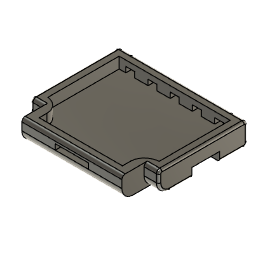
Carcasa Muñeca v1 (Autodesk Fusion 360 design; units mm, degrees)
Autodesk Fusion 360 part; units mm, degrees
sketch "Sketch10" plane through (0, 0, 0) normal (0, 0, 1) x (1, 0, 0)
  line L0 (0, -50) -> (0, 50) construction
  line L1 (0, 50) -> (-57, 50)
  line L2 (-57, 50) -> (-57, 0)
  line L3 (0, -50) -> (-45, -50)
  line L4 (-45, -50) -> (-45, -30)
  arc A0 (-57, 0) -> (-45, -30) centre (-7.0663, 2.5735) ccw
  line L5 (0, -50) -> (45, -50)
  line L6 (45, -50) -> (45, -30)
  arc A1 (45, -30) -> (57, 0) centre (7.0663, 2.5735) ccw
  line L7 (57, 50) -> (57, 0)
  line L8 (0, 50) -> (57, 50)
  dimension "d19" = 100
  dimension "d20" = 57
  dimension "d21" = 50
  dimension "d22" = 45
  dimension "d23" = 20
  dimension "d24" = 50
  dimension "d25" = 30
  constraint vertical L0
  constraint midpoint L0 origin
  constraint perpendicular L0 L1
  constraint perpendicular L1 L2
  constraint perpendicular L0 L3
  constraint perpendicular L3 L4
  constraint symmetric L3.start L0 L5.start
  constraint symmetric L1.start L0 L8.start
  constraint symmetric L0 L1.end L7.start
  constraint symmetric L0 L2.end A1.end
  constraint symmetric L0 L3.end L5.end
  constraint symmetric L0 L4.end L6.end
  constraint symmetric L0 A0 A1
  measures "d19" distance of L0.start L0.end
  measures "d20" distance of L0.end L1.end
  measures "d21" distance of L1.end L2.end
  measures "d22" distance of L0.start L3.end
  measures "d23" distance of L3.end L4.end
  measures "d24" radius of A0
  measures "d25" vertical distance of L2.end L4.end
sketch "Sketch12" plane through (0, 0, 0) normal (1, 0, 0) x (0, 1, 0)
  line L0 (0, 10) -> (0, -10) construction
  line L1 (0, 10) -> (47, 10)
  line L2 (50, 7) -> (50, -7)
  line L3 (47, -10) -> (0, -10)
  arc A0 (50, 7) -> (47, 10) centre (47, 7) ccw
  line L4 (0, 10) -> (-47, 10)
  line L5 (-50, 7) -> (-50, 0)
  line L6 (-40, -10) -> (0, -10)
  arc A1 (-47, 10) -> (-50, 7) centre (-47, 7) ccw
  arc A2 (-50, 0) -> (-40, -10) centre (-40, 0) ccw
  arc A3 (47, -10) -> (50, -7) centre (47, -7) ccw
  dimension "d30" = 3
  dimension "d31" = 47
  dimension "d34" = 3
  dimension "d35" = 10
  dimension "d36" = 7
  dimension "d37" = 40
  dimension "d38" = 3
  dimension "d39" = 47
  dimension "d40" = 14
  constraint vertical L0
  constraint midpoint L0 origin
  constraint perpendicular L0 L1
  constraint perpendicular L1 L2
  constraint tangent L1 A0
  constraint tangent L2 A0
  constraint perpendicular L0 L4
  constraint perpendicular L4 L5
  constraint tangent L5 A1
  constraint tangent L4 A1
  constraint tangent L6 A2
  constraint tangent L5 A2
  constraint tangent L3 A3
  constraint tangent L2 A3
  measures "d30" radius of A0
  measures "d31" distance of L0.start L1.end
  measures "d34" radius of A1
  measures "d35" radius of A2
  measures "d36" distance of L5.start L5.end
  measures "d37" distance of L0.end L6.start
  measures "d38" radius of A3
  measures "d39" distance of L0.end L3.start
  measures "d40" distance of L2.start L2.end
extrude "Extrude1" add sketch "Sketch12" along normal mid plane 90
ref_plane "WorkPlane5" through (-57, 0, 0) normal (-1, 0, 0) x (0, -1, 0)
sketch "Sketch14" plane through (-57, 0, 0) normal (-1, 0, 0) x (0, 1, 0)
ref_plane "WorkPlane6" through (-57, 25, 0) normal (-1, 0, 0) x (0, -1, 0)
sketch "Sketch15" plane through (-57, 25, 0) normal (-1, 0, 0) x (0, 1, 0)
  line L0 (-55, -9.04) -> (-55, -10)
  line L1 (-52, -10) -> (22, -10)
  line L2 (25, -7) -> (25, 7)
  line L3 (22, 10) -> (-45, 10)
  line L4 (-55, 0) -> (-55, -7)
  arc A0 (22, -10) -> (25, -7) centre (22, -7) ccw
  arc A1 (25, 7) -> (22, 10) centre (22, 7) ccw
  line L5 (1.4925, -10) -> (1.4925, 10) construction
  arc A2 (-55, -7) -> (-52, -10) centre (-52, -7) ccw
  arc A3 (-45, 10) -> (-55, 0) centre (-45, 0) ccw
  point P0 (25, 0)
  point P1 (25, 0)
  dimension "d46" = 3
  dimension "d47" = 3
  dimension "d51" = 3
  dimension "d52" = 10
  dimension "d53" = 74
  dimension "d54" = 67
  constraint vertical L0
  constraint perpendicular L0 L1
  constraint perpendicular L1 L2
  constraint perpendicular L2 L3
  constraint tangent L1 A0
  constraint tangent L2 A0
  constraint tangent L2 A1
  constraint tangent L3 A1
  constraint coincident L1 L5.start
  constraint coincident L3 L5.end
  constraint perpendicular L3 L5
  constraint midpoint L2 P1
  constraint coincident P1 P0
  constraint coincident L0.end L1
  constraint coincident L0.start L4
  constraint tangent L1 A2
  constraint tangent L4 A2
  constraint tangent L4 A3
  constraint tangent L3 A3
  measures "d46" radius of A0
  measures "d47" radius of A1
  measures "d51" radius of A2
  measures "d52" radius of A3
  measures "d53" distance of L1.end L1.start
  measures "d54" distance of L3.start L3.end
extrude "Extrude2" add sketch "Sketch15" against normal blind 115
ref_plane "WorkPlane7" through (0.5, 0, 0) normal (0, 0, 1) x (0, -1, 0)
sketch "Sketch16" plane through (0.5, 0, 0) normal (0, 0, 1) x (1, 0, 0)
  line L0 (-57.5, -27) -> (-45.5, -27)
  line L1 (-45.5, 47) -> (-57.5, 47)
  line L2 (44.5, 47) -> (-45.5, 47)
  line L3 (-45.5, -47) -> (44.5, -47)
  line L4 (-50, -22) -> (-49.8646, -22)
  spline S0 degree 3 poles (-38, -34.9844) (-38, -34.1746) (-38.0781, -33.3665) (-38.2356, -32.5653) (-38.4864, -31.2898) (-38.934, -30.0628) (-39.5567, -28.9303) (-40.1006, -27.941) (-40.7649, -27.0442) (-41.5343, -26.2443) (-42.3573, -25.3885) (-43.2746, -24.6713) (-44.259, -24.0826) (-44.6237, -23.8645) (-44.9929, -23.6669) (-45.3645, -23.4878) (-46.062, -23.1516) (-46.7439, -22.8924) (-47.3936, -22.6821) (-47.7428, -22.5691) (-48.0747, -22.4726) (-48.3871, -22.3866) (-48.6995, -22.3007) (-48.9874, -22.2266) (-49.2495, -22.1589) (-49.4545, -22.1059) (-49.6596, -22.053) (-49.8646, -22) knots 0 0 0 0 0.145451 0.145451 0.145451 0.378172 0.378172 0.378172 0.57973 0.57973 0.57973 0.794995 0.794995 0.794995 0.875515 0.875515 0.875515 1.02581 1.02581 1.02581 1.107128 1.107128 1.107128 1.188446 1.188446 1.188446 1.251983 1.251983 1.251983 1.251983
  line L5 (-38, -34.9844) -> (-38, -42)
  line L6 (-38, -42) -> (37, -42)
  line L7 (37, -42) -> (37, -34.9844)
  spline S1 degree 3 poles (48.8646, -22) (48.6596, -22.053) (48.4545, -22.1059) (48.2495, -22.1589) (47.9231, -22.2432) (47.5575, -22.3372) (47.1559, -22.4513) (46.7191, -22.5754) (46.2521, -22.7202) (45.7606, -22.8999) (45.11, -23.1377) (44.4444, -23.427) (43.7768, -23.788) (42.532, -24.4611) (41.372, -25.3353) (40.3642, -26.4246) (39.0898, -27.802) (38.1319, -29.4395) (37.566, -31.2594) (37.189, -32.4721) (37, -33.7198) (37, -34.9844) knots -0.075884 -0.075884 -0.075884 -0.075884 -0.012347 -0.012347 -0.012347 0.088762 0.088762 0.088762 0.198518 0.198518 0.198518 0.343196 0.343196 0.343196 0.611473 0.611473 0.611473 0.950217 0.950217 0.950217 1.176099 1.176099 1.176099 1.176099
  line L8 (48.8646, -22) -> (50, -22)
  line L9 (50, -22) -> (50, 42)
  line L10 (50, 42) -> (44.5, 42)
  line L11 (44.5, 42) -> (-45.5, 42)
  line L12 (-45.5, 42) -> (-50, 42)
  line L13 (-50, 42) -> (-50, -22)
  line L14 (-45.5, -27) -> (-45.5, -47)
  line L15 (44.5, -47) -> (44.5, -27)
  line L16 (-57.5, 47) -> (-57.5, -27)
  line L17 (44.5, -27) -> (57.5, -27)
  line L18 (57.5, -27) -> (57.5, 47)
  line L19 (57.5, 47) -> (44.5, 47)
  constraint parallel L3 L6
  constraint parallel L0 L8
  constraint parallel L1 L10
  constraint parallel L2 L11
extrude "Extrude3" cut sketch "Sketch16" along normal blind 10 contours L4 S0 L5 L6 L7 S1 L8 L9 L10 L11 L12 L13
ref_plane "WorkPlane9" through (58, 13.5, -10) normal (1, 0, 0) x (0, 1, 0)
sketch "Sketch17" plane through (58, 13.5, -10) normal (1, 0, 0) x (0, 1, 0)
  line L0 (-13.5, 0) -> (11.5, 0)
  line L1 (11.5, 0) -> (11.5, 8)
  line L2 (11.5, 8) -> (-13.5, 8)
  line L3 (-13.5, 8) -> (-13.5, 0)
  point P0 (-13.5, 0)
  dimension "d70" = 8
  dimension "d71" = 25
  constraint horizontal L0
  constraint vertical L1
  constraint horizontal L2
  constraint vertical L3
  constraint coincident P0 L0.start
  measures "d70" distance of L0.end L1.end
  measures "d71" distance of P0 L0.end
extrude "Extrude4" cut sketch "Sketch17" against normal blind 15
ref_plane "WorkPlane10" through (50.5, 0, -6) normal (0, 1, 0) x (0, 0, -1)
sketch "Sketch18" plane through (50.5, 0, -6) normal (0, 1, 0) x (1, 0, 0)
  circle A0 centre (0, 0) radius 2.5
  dimension "d75" = 5
  constraint coincident A0.centre origin
  measures "d75" diameter of A0
extrude "Extrude5" add sketch "Sketch18" along normal blind 25
ref_plane "WorkPlane11" through (-57, 10, 0) normal (-1, 0, 0) x (0, 1, 0)
ref_plane "WorkPlane13" through (0.5, 50, 0) normal (0, 1, 0) x (0, 0, 1)
ref_plane "WorkPlane14" through (0.5, 50, 0) normal (0, 1, 0) x (0, 0, 1)
ref_plane "WorkPlane15" through (0, -50, 3.5) normal (0, -1, 0) x (0, 0, -1)
sketch "Sketch24" plane through (0, -50, 3.5) normal (0, -1, 0) x (1, 0, 0)
  line L0 (0, 1.5) -> (0, -3.5) construction
  line L1 (-15, 1.5) -> (15, 1.5)
  line L2 (15, 1.5) -> (15, -3.5)
  line L3 (15, -3.5) -> (-15, -3.5)
  line L4 (-15, -3.5) -> (-15, 1.5)
  line L5 (-15, 1.5) -> (15, -3.5) construction
  line L6 (15, 1.5) -> (-15, -3.5) construction
  point P0 (0, -3.5)
  point P1 (0, -1)
  dimension "d113" = 5
  dimension "d114" = 5
  dimension "d115" = 30
  constraint vertical L0
  constraint coincident P0 L0.end
  constraint horizontal L1
  constraint perpendicular L1 L2
  constraint parallel L1 L3
  constraint parallel L2 L4
  constraint coincident L5 P1
  constraint coincident L6 P1
  constraint midpoint L0 P1
  measures "d113" distance of L0.start P0
  measures "d114" distance of L1.start L3.end
  measures "d115" distance of L1.start L1.end
extrude "Extrude9" cut sketch "Sketch24" against normal blind 8
fillet "Fillet4" radius 2 18 edges at (-57, 13.5, -10) (-57, -27.0711, -7.0711) (-57, -30, 3.5) (-57, -29.1213, 9.1213) (-57, 10, 10) (-57, 49.1213, 9.1213) (-57, 50, 0) (-57, 49.1213, -9.1213) (-57, 13.5, -10) (58, 36, -10) (58, 49.1213, -9.1213) (58, 50, 0) (58, 49.1213, 9.1213) (58, 10, 10) (58, -29.1213, 9.1213) (58, -30, 3.5) (58, -27.0711, -7.0711) (58, -10, -10)
ref_plane "WorkPlane16" through (-57, 10, 0) normal (-1, 0, 0) x (0, 1, 0)
sketch "Sketch25" plane through (-57, 10, 0) normal (-1, 0, 0) x (0, 1, 0)
  line L0 (-10, 10) -> (-10, 2)
  line L1 (15, 2) -> (-10, 2)
  line L2 (-10, 2) -> (-10, 10)
  line L3 (-10, 10) -> (15, 10)
  line L4 (15, 10) -> (15, 2)
  point P0 (-10, 10)
  dimension "d125" = 25
  dimension "d126" = 8
  constraint vertical L0
  constraint horizontal L1
  constraint vertical L2
  constraint horizontal L3
  constraint vertical L4
  constraint coincident P0 L0.start
  measures "d125" distance of L1.start L0.end
  measures "d126" distance of L1.start L3.end
extrude "Extrude10" cut sketch "Sketch25" against normal blind 15
ref_plane "WorkPlane17" through (-49.5, 0, -6) normal (0, 1, 0) x (0, 0, 1)
sketch "Sketch26" plane through (-49.5, 0, -6) normal (0, 1, 0) x (1, 0, 0)
  circle A0 centre (0, 0) radius 2.5
  dimension "d130" = 5
  constraint coincident A0.centre origin
  measures "d130" diameter of A0
extrude "Extrude11" add sketch "Sketch26" along normal blind 25
sketch "Sketch27" plane through (0, 50, 0) normal (0, 1, 0) x (-1, 0, 0)
  line L0 (-56, 7) -> (-56, -7)
  line L1 (-56, -7) -> (-45, -7)
  line L2 (-45, -7) -> (45, -7)
  line L3 (45, -7) -> (55, -7)
  line L4 (55, -7) -> (55, 7)
  line L5 (55, 7) -> (45, 7)
  line L6 (45, 7) -> (-45, 7)
  line L7 (-45, 7) -> (-56, 7)
  line L8 (-56, 0) -> (-44.5, 0) construction
  line L9 (-44.5, 0) -> (-36.5, 0)
  line L10 (-36.5, 0) -> (-36.5, 5)
  line L11 (-36.5, 5) -> (-44.5, 5)
  line L12 (-44.5, 5) -> (-44.5, 0)
  line L13 (-36.5, 0) -> (-24.5, 0) construction
  line L14 (-24.5, 0) -> (-16.5, 0)
  line L15 (-16.5, 0) -> (-16.5, 5)
  line L16 (-16.5, 5) -> (-24.5, 5)
  line L17 (-24.5, 5) -> (-24.5, 0)
  line L18 (-16.5, 0) -> (-4.5, 0) construction
  line L19 (-4.5, 0) -> (3.5, 0)
  line L20 (3.5, 0) -> (3.5, 5)
  line L21 (3.5, 5) -> (-4.5, 5)
  line L22 (-4.5, 5) -> (-4.5, 0)
  line L23 (3.5, 0) -> (15.5, 0) construction
  line L24 (15.5, 0) -> (23.5, 0)
  line L25 (23.5, 0) -> (23.5, 5)
  line L26 (23.5, 5) -> (15.5, 5)
  line L27 (15.5, 5) -> (15.5, 0)
  line L28 (23.5, 0) -> (35.5, 0) construction
  line L29 (35.5, 0) -> (43.5, 0)
  line L30 (43.5, 0) -> (43.5, 5)
  line L31 (43.5, 5) -> (35.5, 5)
  line L32 (35.5, 5) -> (35.5, 0)
  line L33 (43.5, 0) -> (55, 0) construction
  dimension "d134" = 5
  dimension "d135" = 8
  dimension "d136" = 5
  dimension "d137" = 8
  dimension "d138" = 8
  dimension "d139" = 5
  dimension "d140" = 5
  dimension "d141" = 8
  dimension "d142" = 8
  dimension "d143" = 5
  dimension "d144" = 11.5
  dimension "d145" = 12
  dimension "d146" = 12
  dimension "d147" = 12
  dimension "d148" = 12
  dimension "d149" = 11.5
  constraint midpoint L0 L8.start
  constraint perpendicular L0 L8
  constraint horizontal L9
  constraint vertical L10
  constraint horizontal L11
  constraint vertical L12
  constraint perpendicular L10 L13
  constraint horizontal L14
  constraint vertical L15
  constraint horizontal L16
  constraint vertical L17
  constraint perpendicular L15 L18
  constraint horizontal L19
  constraint vertical L20
  constraint horizontal L21
  constraint vertical L22
  constraint perpendicular L20 L23
  constraint horizontal L24
  constraint vertical L25
  constraint horizontal L26
  constraint vertical L27
  constraint perpendicular L25 L28
  constraint horizontal L29
  constraint vertical L30
  constraint horizontal L31
  constraint vertical L32
  constraint midpoint L4 L33.end
  constraint perpendicular L4 L33
  measures "d134" distance of L9.end L10.end
  measures "d135" distance of L10.end L11.end
  measures "d136" distance of L13.end L16.end
  measures "d137" distance of L15.end L16.end
  measures "d138" distance of L20.end L21.end
  measures "d139" distance of L18.end L21.end
  measures "d140" distance of L23.end L26.end
  measures "d141" distance of L25.end L26.end
  measures "d142" distance of L30.end L31.end
  measures "d143" distance of L28.end L31.end
  measures "d144" distance of L8.start L8.end
  measures "d145" distance of L9.end L13.end
  measures "d146" distance of L14.end L18.end
  measures "d147" distance of L19.end L23.end
  measures "d148" distance of L24.end L28.end
  measures "d149" distance of L29.end L33.end
extrude "Extrude12" cut sketch "Sketch27" against normal blind 8 contours L9 L10 L11 L12 | L14 L15 L16 L17 | L19 L20 L21 L22 | L24 L25 L26 L27 | L29 L30 L31 L32
sketch "Sketch28" plane through (-3.5, 0, 0) normal (1, 0, 0) x (0, 1, 0)
move_body "Move1" bodies 1 to x (1, 0, 0) y (0, 1, 0) z (0, 0, 1) at (-7.4393, -88.2855, 0)
scale "Scale1" factor 0.6 about (-22.9393, -46.2855, 0) bodies 1
move_body "Move2" bodies 1 to x (1, 0, 0) y (0, 1, 0) z (0, 0, 1) at (-1.064, -13.1586, 0)
